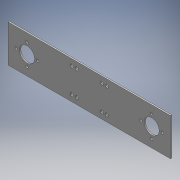
# Autodesk Inventor part: UpperArm2
Saved by Autodesk Inventor 2016 (Build 200138000, 138)
## iProperties
Created: 2016-06-25
Part Number: UpperArm2
Material: 一般
Document SubType Name: Modeling
Designer: 宏太
Density: 1 g/cm^3
Appearance: 既定
Mass: 115.316 g
Surface Area: 370.453 cm^2
Volume: 115.316 cm^3
Author: 宏太
Autodesk Inventor part; units mm, degrees
ref_plane "YZ Plane" through (0, 0, 0) normal (1, 0, 0) x (0, 1, 0)
ref_plane "XZ Plane" through (0, 0, 0) normal (0, 1, 0) x (-1, 0, 0)
ref_plane "XY Plane" through (0, 0, 0) normal (0, 0, 1) x (1, 0, 0)
sketch "スケッチ1" plane through (0, 0, 0) normal (0, 1, 0) x (-1, 0, 0)
  line L0 (-130, -30) -> (130, -30)
  line L1 (130, -30) -> (130, 30)
  line L2 (130, 30) -> (-130, 30)
  line L3 (-130, 30) -> (-130, -30)
  line L4 (-130, -30) -> (130, 30) construction
  line L5 (130, -30) -> (-130, 30) construction
  circle A0 centre (-28, -20) radius 2.6
  circle A1 centre (-20, -20) radius 2.6
  circle A2 centre (20, -20) radius 2.6
  circle A3 centre (28, -20) radius 2.6
  circle A4 centre (-28, 20) radius 2.6
  circle A5 centre (-20, 20) radius 2.6
  circle A6 centre (20, 20) radius 2.6
  circle A7 centre (28, 20) radius 2.6
  point P0 (0, 0)
  dimension "d0" = 260
  dimension "d1" = 60
  dimension "d2" = 5.2
  dimension "d4" = 5.2
  dimension "d5" = 8
  dimension "d6" = 5.2
  dimension "d7" = 40
  dimension "d8" = 5.2
  dimension "d9" = 8
  dimension "d10" = 5.2
  dimension "d12" = 5.2
  dimension "d13" = 5.2
  dimension "d14" = 5.2
  dimension "d16" = 40
  dimension "d17" = 8
  dimension "d18" = 8
  dimension "d20" = 10
  dimension "d21" = 158
  dimension "d22" = 50
  dimension "d23" = 158
  constraints: 12 end point, 8 centre point, 2 midpoint, 2 parallel, 1 horizontal, 1 perpendicular
  measures "d0" distance of L2.end L1.end
  measures "d1" distance of L1.end L0.end
  measures "d2" diameter of A0
  measures "d4" diameter of A1
  measures "d5" distance of A1.centre A0.centre
  measures "d6" diameter of A2
  measures "d7" distance of A2.centre A1.centre
  measures "d8" diameter of A3
  measures "d9" distance of A3.centre A2.centre
  measures "d10" diameter of A4
  measures "d12" diameter of A5
  measures "d13" diameter of A6
  measures "d14" diameter of A7
  measures "d16" distance of A6.centre A5.centre
  measures "d17" distance of A7.centre A6.centre
  measures "d18" distance of A5.centre A4.centre
  measures "d20" distance from line of L0 A0.centre
  measures "d21" distance from line of L3 A3.centre
  measures "d22" distance from line of L0 A4.centre
  measures "d23" distance from line of L3 A7.centre
extrude "押し出し1" add sketch "スケッチ1" along normal blind 2
sketch "スケッチ2" plane through (0, 0, 0) normal (0, -1, 0) x (1, 0, 0)
  circle A0 centre (-100, 0) radius 12
  circle A1 centre (100, 0) radius 12
  line L0 (-130, -30) -> (-130, 30) projected
  line L1 (130, 30) -> (130, -30) projected
  point P0 (0, 0)
  dimension "d26" = 24
  dimension "d27" = 24
  dimension "d28" = 30
  dimension "d29" = 30
  constraints: 2 centre point
  measures "d26" diameter of A0
  measures "d27" diameter of A1
  measures "d28" distance from line of L0 A0.centre
  measures "d29" distance from line of L1 A1.centre
extrude "押し出し2" cut sketch "スケッチ2" against normal blind 10
sketch "スケッチ3" plane through (0, 0, 0) normal (0, -1, 0) x (1, 0, 0)
  circle A0 centre (-100, 0) radius 12 projected
  circle A1 centre (-100, 17) radius 2.1
  circle A2 centre (-83, 0) radius 2.1
  circle A3 centre (-100, -17) radius 2.1
  circle A4 centre (-117, 0) radius 2.1
  circle A5 centre (100, 0) radius 12 projected
  circle A6 centre (100, 17) radius 2.1
  circle A7 centre (117, 0) radius 2.1
  circle A8 centre (83, 0) radius 2.1
  circle A9 centre (100, -17) radius 2.1
  point P0 (0, 0)
  dimension "d33" = 4.2
  dimension "d34" = 4.2
  dimension "d35" = 4.2
  dimension "d36" = 4.2
  dimension "d38" = 4.2
  dimension "d39" = 4.2
  dimension "d40" = 4.2
  dimension "d41" = 4.2
  constraints: 8 centre point
  measures "d33" diameter of A1
  measures "d34" diameter of A2
  measures "d35" diameter of A3
  measures "d36" diameter of A4
  measures "d38" diameter of A6
  measures "d39" diameter of A7
  measures "d40" diameter of A8
  measures "d41" diameter of A9
extrude "押し出し3" cut sketch "スケッチ3" against normal blind 10 contours A1 | A2 | A3 | A4 | A6 | A7 | A8 | A9
